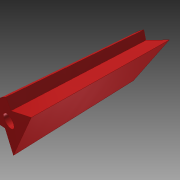
# Autodesk Inventor part: filament_guide_spool
Saved by Autodesk Inventor 2014 (Build 180170000, 170)
## iProperties
Created: 2014-04-06
Part Number: filament_guide_spool
Material: ABS Plastic
Document SubType Name: Modeling
Designer: buben
Density: 1.06 g/cm^3
Appearance: Light Red
Author: buben
Autodesk Inventor part; units mm, degrees
ref_plane "YZ Plane" through (0, 0, 0) normal (1, 0, 0) x (0, 1, 0)
ref_plane "XZ Plane" through (0, 0, 0) normal (0, 1, 0) x (-1, 0, 0)
ref_plane "XY Plane" through (0, 0, 0) normal (0, 0, 1) x (1, 0, 0)
sketch "Sketch1" plane through (0, 0, 0) normal (0, 1, 0) x (-1, 0, 0)
  circle A0 centre (0, 0) radius 4.2
  line L0 (11.4529, -8.6044) -> (5.0517, -7.4757) construction
  line L1 (5.0517, -7.4757) -> (-4.499, -61.6402) construction
  line L2 (-4.499, -61.6402) -> (1.9023, -62.7689) construction
  line L3 (1.9023, -62.7689) -> (11.4529, -8.6044) construction
  line L4 (-3.9483, 8.1127) -> (-1.7252, 14.2207) construction
  line L5 (-1.7252, 14.2207) -> (-53.4083, 33.0318) construction
  line L6 (-53.4083, 33.0318) -> (-55.6314, 26.9238) construction
  line L7 (-55.6314, 26.9238) -> (-3.9483, 8.1127) construction
  arc A1 (11.4529, -8.6044) -> (-1.7252, 14.2207) centre (-10.3924, -6.0001) ccw
  line L8 (-3.9483, 8.1127) -> (-55.6314, 8.1127) construction
  line L9 (5.0517, -7.4757) -> (-3.9483, 8.1127) construction
  line L10 (0.5517, 0.3185) -> (-10.3924, -6.0001) construction
  line L11 (2.1781, -23.7726) -> (-19.4986, 13.7726)
  line L12 (11.4529, -8.6044) -> (5.0517, -7.4757)
  line L13 (5.0517, -7.4757) -> (2.1781, -23.7726)
  line L14 (-19.4986, 13.7726) -> (-3.9483, 8.1127)
  line L15 (-3.9483, 8.1127) -> (-1.7252, 14.2207)
  dimension "d0" = 8.4
  dimension "d2" = 6.5
  dimension "d3" = 55
  dimension "d4" = 100
  dimension "d5" = 22
  dimension "d6" = 18
  dimension "d7" = 20
  dimension "d8" = 0.637
  dimension "d9" = 10
  constraints: 32 end point, 5 perpendicular, 4 parallel, 3 collinear, 3 point on line, 2 centre point, 2 equal length, 2 point on circle, 1 coincident, 1 horizontal, 1 midpoint, 1 vertical alignment
  measures "d0" diameter of A0
  measures "d2" distance of L0.start L0.end
  measures "d3" distance of L2.end L0.start
  measures "d4" angle of L7 L1
  measures "d5" radius of A1
  measures "d6" distance of L4.start L0.end
  measures "d7" angle of L7 L8
  measures "d8" distance of L10.start point (0, 0)
  measures "d9" distance from line of L11 point (0, 0)
extrude "Extrusion1" add sketch "Sketch1" along normal blind 95
body "Solid1"
